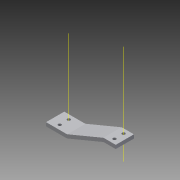
# Autodesk Inventor part: Y_shaft_support_brace_B
Saved by Autodesk Inventor 2013 (Build 170138000, 138)
## iProperties
Created: 2013-09-23
Part Number: Y_shaft_support_brace_B
Material: Aluminum 6061
Document SubType Name: Modeling
Designer: Ian
Density: 2.71 g/cm^3
Mass: 111.844 g
Surface Area: 147.353 cm^2
Volume: 41.2708 cm^3
d8: 0.300 in
d9: 0.300 in
d13: 5.735 in
d21: 1.500 in
d22: 0.225 in
d23: 1.725 in
d24: 3.010 in
d26: 0.300 in
d27: 1.500 in
d28: 0.00 deg
d29: 0.250 in
d30: 0.375 in
d31: 0.375 in
d32: 0.750 in
d33: 0.375 in
d34: 0.375 in
d35: 0.257 in
d42: 0.257 in
d49: 1.250 in
d25: 1.000 in
Author: Ian
Autodesk Inventor part; units mm, degrees
ref_plane "YZ Plane" through (0, 0, 0) normal (1, 0, 0) x (0, 1, 0)
ref_plane "XZ Plane" through (0, 0, 0) normal (0, 1, 0) x (-1, 0, 0)
ref_plane "XY Plane" through (0, 0, 0) normal (0, 0, 1) x (1, 0, 0)
sketch "Sketch1" plane through (0, 0, 0) normal (0, 0, 1) x (1, 0, 0)
  line L0 (5.715, 0) -> (82.169, 31.75)
  line L1 (82.169, 31.75) -> (107.569, 31.75)
  line L2 (107.569, 31.75) -> (107.569, 24.13)
  line L3 (107.569, 24.13) -> (82.169, 24.13)
  line L4 (82.169, 24.13) -> (5.715, -7.62)
  line L5 (5.715, -7.62) -> (-38.1, -7.62)
  line L6 (-38.1, 0) -> (-38.1, -7.62)
  line L7 (-38.1, 0) -> (5.715, 0)
  point P0 (0, 0)
  dimension "d8" = 7.62
  dimension "d9" = 7.62
  dimension "d13" = 145.669
  dimension "d21" = 38.1
  dimension "d22" = 5.715
  dimension "d23" = 43.815
  dimension "d24" = 76.454
  dimension "d25" = 25.4
  dimension "d26" = 7.62
  dimension "d49" = 31.75
  constraints: 16 end point, 4 parallel, 2 perpendicular, 1 vertical
  measures "d8" distance of L5.end L6.start
  measures "d9" distance of L1.end L2.end
  measures "d13" distance between parallel lines of L2 L6
  measures "d21" distance of L6.start point (0, 0)
  measures "d22" distance of point (0, 0) L0.start
  measures "d23" distance of L5.end L4.end
  measures "d24" horizontal distance of L3.end L4.end
  measures "d25" distance of L2.end L3.end
  measures "d26" distance of L0.start L4.end
  measures "d49" vertical distance of L0.start L0.end
extrude "Extrusion1" add sketch "Sketch1" along normal blind 38.1
fillet "Fillet1" radius 6.35 4 edges at (5.715, -7.62, 19.05) (5.715, 0, 19.05) (82.169, 31.75, 19.05) (82.169, 24.13, 19.05)
sketch "Sketch2" plane through (107.569, 24.13, 0) normal (0, -1, 0) x (1, 0, 0)
  line L0 (-24.1339, 0) -> (-24.1339, 38.1) projected
  line L1 (-24.1339, 0) -> (0, 0) projected
  line L2 (0, 0) -> (0, 38.1) projected
  line L3 (-24.1339, 38.1) -> (0, 38.1) projected
  line L4 (-12.0669, 38.1) -> (-12.0669, 0) construction
  line L5 (0, 19.05) -> (-24.1339, 19.05) construction
  point P0 (-107.569, 0)
  point P1 (-12.0669, 9.525)
  point P2 (-12.0669, 28.575)
  dimension "d30" = 9.525
  dimension "d31" = 9.525
  constraints: 4 end point, 4 midpoint, 2 point on line
  measures "d30" distance from line of L3 point (-12.067, 28.575)
  measures "d31" distance from line of L1 point (-12.067, 9.525)
sketch "Sketch3" plane through (-38.1, -7.62, 0) normal (0, -1, 0) x (1, 0, 0)
  line L0 (0, 38.1) -> (42.5489, 38.1) projected
  line L1 (0, 0) -> (0, 38.1) projected
  line L2 (0, 0) -> (42.5489, 0) projected
  line L3 (19.05, 38.1) -> (19.05, 0)
  point P0 (38.1, 0)
  point P1 (19.05, 28.575)
  point P2 (19.05, 9.525)
  dimension "d32" = 19.05
  dimension "d33" = 9.525
  dimension "d34" = 9.525
  constraints: 4 point on line, 2 end point, 1 perpendicular
  measures "d32" distance between parallel lines of L1 L3
  measures "d33" distance from line of L2 point (19.05, 9.525)
  measures "d34" distance from line of point (19.05, 28.575) L0
hole "Hole1" at (95.5021, 24.13, 28.575) at (95.5021, 24.13, 9.525) direction (0, 1, 0) diameter 6.5278 end through all clearance for "Flat Head Machine Screw (82)" size "1/4" standard "Ansi Unified Screw Threads"
hole "Hole2" at (-19.05, -7.62, 28.575) at (-19.05, -7.62, 9.525) direction (0, 1, 0) diameter 6.5278 end through all clearance for "Flat Head Machine Screw (82)" size "1/4" standard "Ansi Unified Screw Threads"
equation "\"d31\" = d30"
equation "\"d34\" = d33"
body "Solid1"
